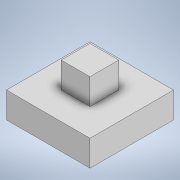
# Autodesk Inventor part: Motor_fit_check
Saved by Autodesk Inventor 2022 (Build 260153000, 153)
## iProperties
Created: 2023-02-21
Part Number: Motor_fit_check
Material: Generic
Document SubType Name: Modeling
Designer: zarek
Density: 1 g/cm^3
Appearance: Default
Author: zarek
Autodesk Inventor part; units mm, degrees
ref_plane "YZ Plane" through (0, 0, 0) normal (1, 0, 0) x (0, 1, 0)
ref_plane "XZ Plane" through (0, 0, 0) normal (0, 1, 0) x (-1, 0, 0)
ref_plane "XY Plane" through (0, 0, 0) normal (0, 0, 1) x (1, 0, 0)
sketch "Sketch1" plane through (0, 0, 0) normal (0, 1, 0) x (-1, 0, 0)
  line L0 (14.5, -14.5) -> (-14.5, -14.5)
  line L1 (-14.5, -14.5) -> (-14.5, 14.5)
  line L2 (-14.5, 14.5) -> (14.5, 14.5)
  line L3 (14.5, 14.5) -> (14.5, -14.5)
  dimension "d11" = 29
  dimension "d14" = 29
  constraints: 8 end point, 2 parallel, 1 horizontal, 1 perpendicular
  measures "d11" distance between parallel lines of L1 L3
  measures "d14" distance between parallel lines of L2 L0
extrude "Extrusion1" add sketch "Sketch1" along normal blind 9
sketch "Sketch2" plane through (0, 9, 0) normal (0, 1, 0) x (1, 0, 0)
  line L0 (-5, 5) -> (5, 5)
  line L1 (5, 5) -> (5, -5)
  line L2 (5, -5) -> (-5, -5)
  line L3 (-5, -5) -> (-5, 5)
  line L4 (14.5, 14.5) -> (-14.5, 14.5) projected
  line L5 (14.5, -14.5) -> (14.5, 14.5) projected
  line L6 (-14.5, -14.5) -> (14.5, -14.5) projected
  line L7 (-14.5, 14.5) -> (-14.5, -14.5) projected
  point P0 (0, 0)
  dimension "d15" = 9.5
  dimension "d16" = 9.5
  dimension "d17" = 9.5
  dimension "d18" = 9.5
  constraints: 8 end point, 2 parallel, 1 horizontal, 1 perpendicular
  measures "d15" distance between parallel lines of L0 L4
  measures "d16" distance between parallel lines of L5 L1
  measures "d17" distance between parallel lines of L6 L2
  measures "d18" distance between parallel lines of L7 L3
extrude "Extrusion2" add sketch "Sketch2" along normal blind 9 contours L0 L1 L2 L3
sketch "Sketch3" plane through (0, 0, 0) normal (0, -1, 0) x (1, 0, 0)
  line L0 (2.54, 1.778) -> (-2.54, 1.778)
  line L1 (-2.794, 1.524) -> (-2.794, -1.524)
  line L2 (-2.54, -1.778) -> (2.54, -1.778)
  line L3 (2.794, -1.524) -> (2.794, 1.524)
  arc A0 (2.794, 1.7526) -> (2.7686, 1.778) centre (2.7686, 1.7526) ccw
  arc A1 (2.794, 1.524) -> (2.54, 1.778) centre (2.54, 1.524) ccw
  arc A2 (2.54, -1.778) -> (2.794, -1.524) centre (2.54, -1.524) ccw
  arc A3 (-2.794, -1.524) -> (-2.54, -1.778) centre (-2.54, -1.524) ccw
  arc A4 (-2.54, 1.778) -> (-2.794, 1.524) centre (-2.54, 1.524) ccw
  point P0 (0, 0)
  point P1 (-0.254, 0)
  point P2 (-0.254, 0)
  dimension "d21" = 1.778
  dimension "d22" = 3.556
  dimension "d23" = 5.588
  dimension "d24" = 2.54
  dimension "d25" = 0.0254
  dimension "d26" = 0.254
  dimension "d27" = 2.794
  dimension "d28" = 1.778
  constraints: 10 point on circle, 10 tangent, 8 end point, 5 centre point, 3 equal radius, 2 parallel, 2 point on line, 1 coincident, 1 horizontal, 1 perpendicular
  measures "d21" distance from line of point (-0.254, 0) L0
  measures "d22" distance between parallel lines of L2 L0
  measures "d23" distance between parallel lines of L1 L3
  measures "d24" distance from line of L1 point (-0.254, 0)
  measures "d25" radius of A0
  measures "d26" radius of A1
  measures "d27" distance from line of L3 point (0, 0)
  measures "d28" distance from line of L2 point (0, 0)
extrude "Extrusion3" cut sketch "Sketch3" against normal blind 6
sketch "Sketch4" plane through (0, 0, 0) normal (0, -1, 0) x (1, 0, 0)
  point P0 (0, 0)
equation "\"d14\" = d11"
equation "\"d16\" = d15"
equation "\"d17\" = d15"
equation "\"d18\" = d15"
equation "\"d21\" = 0.5 * d22"
body "Solid1"
